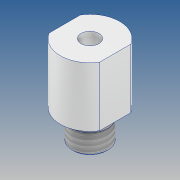
# Autodesk Inventor part: 102.002.01_Justage_Vereinzelung
Saved by Autodesk Inventor 2021 (Build 250183000, 183)
## iProperties
Created: 2021-11-26
Part Number: 102.002.01_Justage_Vereinzelung
Material: Aluminium 6061
Document SubType Name: Modeling
Designer: Oliver Ungerer
Density: 2.7 g/cm^3
Appearance: Aluminium - flach
Mass: 16.319 g
Surface Area: 27.2754 cm^2
Volume: 6.04408 cm^3
Author: Oliver Ungerer
Title: Justageschraube
Autodesk Inventor part; units mm, degrees
ref_plane "YZ Plane" through (0, 0, 0) normal (1, 0, 0) x (0, 1, 0)
ref_plane "XZ Plane" through (0, 0, 0) normal (0, 1, 0) x (-1, 0, 0)
ref_plane "XY Plane" through (0, 0, 0) normal (0, 0, 1) x (1, 0, 0)
sketch "Skizze6" plane through (0, 0, 0) normal (0, 0, 1) x (1, 0, 0)
  line L0 (0, 0) -> (6, 0)
  line L1 (6, 0) -> (6, 10)
  line L2 (6, 10) -> (10, 10)
  line L3 (10, 10) -> (10, 30)
  line L4 (10, 30) -> (0, 30)
  line L5 (0, 30) -> (0, 0)
  line L6 (0, 30) -> (0, 0)
  dimension "d34" = 20
  dimension "d35" = 12
  dimension "d36" = 20
  dimension "d37" = 30
  constraints: 14 end point, 4 perpendicular, 1 collinear, 1 horizontal, 1 vertical
  measures "d34" diameter of L3 L5
  measures "d35" diameter of L1 L5
  measures "d36" distance between parallel lines of L4 L2
  measures "d37" distance between parallel lines of L0 L4
revolve "Umdrehung1" add sketch "Skizze6" angle 360 about axis through (0, 30, 0) along (0, -1, 0)
sketch "Skizze7" plane through (0, 30, 0) normal (0, 1, 0) x (1, 0, 0)
  circle A0 centre (0, 0) radius 10 projected
  constraints: 1 coincident
hole "Bohrung5" at (0, 30, 0) direction (0, -1, 0) diameter 6 end through all
sketch "Skizze8" plane through (0, 30, 0) normal (0, 1, 0) x (1, 0, 0)
  line L0 (-8.5, -5.2678) -> (-8.5, 5.2678)
  circle A0 centre (0, 0) radius 10 projected
  line L1 (0, 10) -> (0, -10)
  arc A1 (-8.5, 5.2678) -> (-8.5, -5.2678) centre (0, 0) ccw
  line L2 (8.5, -5.2678) -> (8.5, 5.2678)
  arc A2 (8.5, -5.2678) -> (8.5, 5.2678) centre (0, 0) ccw
  dimension "d46" = 17
  constraints: 8 point on circle, 6 end point, 2 centre point, 2 symmetric about line, 2 vertical, 1 concentric, 1 midpoint, 1 other
  measures "d46" diameter of L0 L1
extrude "Extrusion2" cut sketch "Skizze8" against normal up to surface (20 mm away) contours A0 L0 | L2 A0
chamfer "Fase1" distance 0.5 angle 45 1 edges at (-6, 0, 0)
sketch "Skizze9" plane through (0, 0, 0) normal (1, 0, 0) x (0, 1, 0)
  line L0 (10, 6) -> (0.5, 6) projected
  line L1 (10, -5.2678) -> (10, 5.2678) projected
  line L2 (10, 6) -> (10, 4.75)
  line L3 (10, 5.2678) -> (10, -5.2678) projected
  line L4 (10, 4.75) -> (9, 4.75)
  line L5 (9, 4.75) -> (6.8349, 6)
  line L6 (6.8349, 6) -> (10, 6)
  line L7 (0, 0) -> (30, 0)
  line L8 (30, 3) -> (30, -3) projected
  dimension "d52" = 9.5
  dimension "d53" = 30
  dimension "d54" = 1
  constraints: 10 end point, 2 point on line, 1 horizontal, 1 midpoint, 1 parallel
  measures "d52" diameter of L4 L7
  measures "d53" angle of L0 L5
  measures "d54" distance from line of L4.end L1
revolve "Umdrehung2" cut sketch "Skizze9" angle 360 about axis through (0, 0, 0) along (0, 1, 0)
fillet "Rundung1" radius 0.3 2 edges at (0, 10, -4.75) (0, 9, -4.75)
thread "Gewinde1" size "M12x1.75" class "6g" standard "ANSI Metric M Profile" full length
